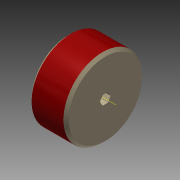
# Autodesk Inventor part: Wheel Temp
Saved by Autodesk Inventor 2013 (Build 170138000, 138)
## iProperties
Created: 2013-06-04
Part Number: Wheel Temp
Material: Generic
Document SubType Name: Modeling
Designer: mvarma
Density: 1 g/cm^3
Author: mvarma
Autodesk Inventor part; units mm, degrees
ref_plane "YZ Plane" through (0, 0, 0) normal (1, 0, 0) x (0, 1, 0)
ref_plane "XZ Plane" through (0, 0, 0) normal (0, 1, 0) x (-1, 0, 0)
ref_plane "XY Plane" through (0, 0, 0) normal (0, 0, 1) x (1, 0, 0)
sketch "Sketch1" plane through (0, 0, 0) normal (0, 0, 1) x (1, 0, 0)
  line L0 (0, 0) -> (44.45, 0)
  line L1 (44.45, 0) -> (44.45, 46.99)
  line L2 (44.45, 46.99) -> (0, 46.99)
  line L3 (0, 46.99) -> (0, 0)
  dimension "d0" = 46.99
  dimension "d1" = 44.45
  constraints: 8 end point, 2 parallel, 1 horizontal, 1 perpendicular
  measures "d0" distance of L2.end L0.start
  measures "d1" distance of L0.start L0.end
revolve "Revolution1" add sketch "Sketch1" angle 360 about axis through (0, 0, 0) along (1, 0, 0)
chamfer "Chamfer1" distance 3.175 angle 45 2 edges at (44.45, -46.99, 0) (0, -46.99, 0)
sketch "Sketch2" plane through (44.45, 0, 0) normal (1, 0, 0) x (0, 0, -1)
  circle A0 centre (0, 0) radius 43.815 projected
  line L0 (6.4158, 0) -> (3.2079, -5.5562)
  line L1 (3.2079, -5.5562) -> (-3.2079, -5.5562)
  line L2 (-3.2079, -5.5562) -> (-6.4158, 0)
  line L3 (-6.4158, 0) -> (-3.2079, 5.5563)
  line L4 (-3.2079, 5.5563) -> (3.2079, 5.5563)
  line L5 (3.2079, 5.5563) -> (6.4158, 0)
  dimension "d6" = 11.1125
  constraints: 12 end point, 1 coincident, 1 horizontal, 13 other
  measures "d6" distance between parallel lines of L1 L4
extrude "Extrusion1" cut sketch "Sketch2" against normal through all contours L0 L1 L2 L3 L4 L5
body "Solid1"
